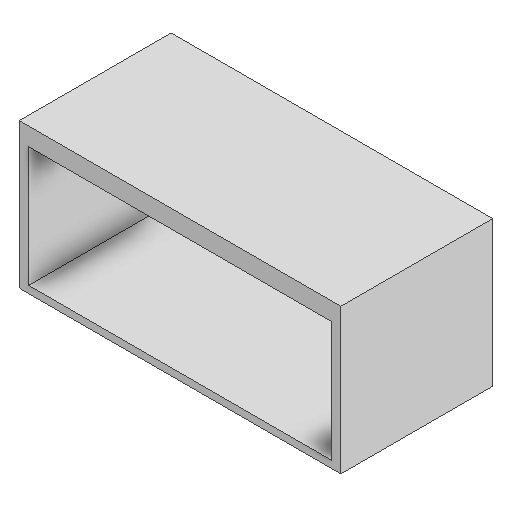
# Autodesk Inventor part: Liv Mas Base Box
Saved by Autodesk Inventor 2025.1 (Build 291241020, 241B)
## iProperties
Created: 2024-03-03
Part Number: Liv Mas Base Box
Material: Generic
Document SubType Name: Modeling
Designer: alexa_e021yt5
Density: 1 g/cm^3
Appearance: Default
Author: alexa_e021yt5
Autodesk Inventor part; units mm, degrees
ref_plane "YZ Plane" through (0, 0, 0) normal (1, 0, 0) x (0, 1, 0)
ref_plane "XZ Plane" through (0, 0, 0) normal (0, 1, 0) x (-1, 0, 0)
ref_plane "XY Plane" through (0, 0, 0) normal (0, 0, 1) x (1, 0, 0)
sketch "Sketch1" plane through (0, 0, 0) normal (0, 0, 1) x (1, 0, 0)
  line L0 (6.35, -116.84) -> (8.89, -119.38)
  line L1 (8.89, -119.38) -> (8.89, -121.92)
  line L2 (6.35, -84.074) -> (6.35, -116.84)
  line L3 (8.89, -81.534) -> (6.35, -84.074)
  line L4 (8.89, -68.58) -> (8.89, -81.534)
  line L5 (74.93, -68.58) -> (8.89, -68.58)
  line L6 (74.93, -121.92) -> (74.93, -68.58)
  line L7 (8.89, -121.92) -> (74.93, -121.92)
  line L8 (5.334, -117.2608) -> (7.874, -119.8008)
  line L9 (7.874, -119.8008) -> (7.874, -122.936)
  line L10 (7.874, -122.936) -> (75.946, -122.936)
  line L11 (75.946, -122.936) -> (75.946, -67.564)
  line L12 (75.946, -67.564) -> (7.874, -67.564)
  line L13 (7.874, -67.564) -> (7.874, -81.1132)
  line L14 (7.874, -81.1132) -> (5.334, -83.6532)
  line L15 (5.334, -83.6532) -> (5.334, -117.2608)
  line L16 (0, -63.5) -> (81.28, -63.5)
  line L17 (81.28, -63.5) -> (81.28, 0)
  line L18 (81.28, 0) -> (0, 0)
  line L19 (0, 0) -> (0, -63.5)
  line L20 (5.334, -111.1172) -> (0, -111.1172) construction
  line L21 (75.946, -101.4463) -> (81.28, -101.4463) construction
  line L22 (34.5139, -122.936) -> (34.5139, -63.5) construction
  line L23 (37.8868, -59.436) -> (37.8868, 0) construction
  line L24 (75.946, -76.28) -> (81.28, -76.28)
  line L25 (75.946, -120.595) -> (81.28, -120.595)
  line L26 (75.946, -107.895) -> (81.28, -107.895)
  line L27 (75.946, -91.52) -> (79.6093, -91.52)
  line L28 (81.28, -89.46) -> (81.28, -78.34)
  line L29 (76.835, -110.245) -> (76.835, -118.245)
  circle A0 centre (8.89, -114.3) radius 1.5875
  circle A1 centre (60.96, -119.38) radius 1.5875
  circle A2 centre (59.69, -71.12) radius 1.5875
  circle A3 centre (8.89, -86.36) radius 1.5875
  circle A4 centre (8.89, -114.3) radius 1.0795
  circle A5 centre (8.89, -86.36) radius 1.0795
  circle A6 centre (59.69, -71.12) radius 1.0795
  circle A7 centre (60.96, -119.38) radius 1.0795
  circle A8 centre (40.64, -95.2527) radius 8.89
  line L30 (6.35, -10.16) -> (8.89, -7.62)
  line L31 (8.89, -7.62) -> (8.89, -5.08)
  line L32 (6.35, -42.926) -> (6.35, -10.16)
  line L33 (8.89, -45.466) -> (6.35, -42.926)
  line L34 (8.89, -58.42) -> (8.89, -45.466)
  line L35 (74.93, -58.42) -> (8.89, -58.42)
  line L36 (74.93, -5.08) -> (74.93, -58.42)
  line L37 (8.89, -5.08) -> (74.93, -5.08)
  line L38 (5.334, -9.7392) -> (7.874, -7.1992)
  line L39 (7.874, -7.1992) -> (7.874, -4.064)
  line L40 (7.874, -4.064) -> (75.946, -4.064)
  line L41 (75.946, -4.064) -> (75.946, -59.436)
  line L42 (75.946, -59.436) -> (7.874, -59.436)
  line L43 (7.874, -59.436) -> (7.874, -45.8868)
  line L44 (7.874, -45.8868) -> (5.334, -43.3468)
  line L45 (5.334, -43.3468) -> (5.334, -9.7392)
  line L46 (5.334, -15.8828) -> (0, -15.8828) construction
  line L47 (75.946, -25.5537) -> (81.28, -25.5537) construction
  line L48 (75.946, -50.72) -> (81.28, -50.72)
  line L49 (75.946, -6.405) -> (81.28, -6.405)
  line L50 (75.946, -19.105) -> (81.28, -19.105)
  line L51 (75.946, -35.48) -> (81.28, -35.48)
  line L52 (81.28, -37.54) -> (81.28, -48.66)
  line L53 (76.835, -16.755) -> (76.835, -8.755)
  circle A9 centre (8.89, -12.7) radius 1.5875
  circle A10 centre (60.96, -7.62) radius 1.5875
  circle A11 centre (59.69, -55.88) radius 1.5875
  circle A12 centre (8.89, -40.64) radius 1.5875
  circle A13 centre (8.89, -12.7) radius 1.0795
  circle A14 centre (8.89, -40.64) radius 1.0795
  circle A15 centre (59.69, -55.88) radius 1.0795
  circle A16 centre (60.96, -7.62) radius 1.0795
  circle A17 centre (40.64, -31.7473) radius 8.89
  point P0 (0, 0)
  point P1 (81.28, -130.1977)
  point P2 (77.7776, -91.52)
  point P3 (81.28, -83.9)
  point P4 (76.835, -114.245)
  point P5 (8.89, -120.65)
  point P6 (41.91, -121.92)
  point P7 (81.28, 3.1977)
  point P8 (34.5139, -4.064)
  point P9 (79.6093, -35.48)
  point P10 (77.7776, -35.48)
  point P11 (81.28, -43.1)
  point P12 (76.835, -12.755)
  point P13 (8.89, -6.35)
  point P14 (41.91, -5.08)
  dimension "d0" = 1.016
  dimension "d1" = 81.28
  dimension "d2" = 63.5
  dimension "d3" = 15.24
  dimension "d4" = 7.62
  dimension "d5" = 12.7
  dimension "d6" = 6.35
  dimension "d7" = 2.159
  dimension "d8" = 2.159
  dimension "d9" = 2.159
  dimension "d10" = 2.159
  dimension "d38" = 17.78
  dimension "d40" = 40.64
  dimension "d93" = 5.334
  dimension "d94" = 63.5
  dimension "d96" = 55.372
  dimension "d97" = 4.064
  dimension "d98" = 4.6592
  dimension "d99" = 2.54
  dimension "d100" = 12.954
  dimension "d101" = 12.5332
  dimension "d102" = 15.0732
  dimension "d103" = 15.494
  dimension "d104" = 6.35
  dimension "d105" = 35.56
  dimension "d106" = 2.54
  dimension "d107" = 50.8
  dimension "d108" = 6.1261
  dimension "d109" = 1.27
  dimension "d110" = 26.6673
  constraints: 108 end point, 44 symmetric about line, 18 centre point, 16 point on line, 9 perpendicular, 5 midpoint, 4 parallel, 1 horizontal, 16 other
  measures "d0" distance between parallel lines of L15 L2
  measures "d1" distance between parallel lines of L17 L19
  measures "d2" distance between parallel lines of L16 L18
  measures "d3" distance from line of point (77.778, -91.52) L24
  measures "d4" distance from line of point (81.28, -83.9) L24
  measures "d5" distance between parallel lines of L25 L26
  measures "d6" distance from line of point (76.835, -114.245) L25
  measures "d7" diameter of A4
  measures "d8" diameter of A7
  measures "d9" diameter of A6
  measures "d10" diameter of A5
  measures "d38" diameter of A8
  measures "d40" distance from line of A8.centre L19
  measures "d93" distance of L20.start L20.end
  measures "d94" distance from line of point (0, 0) L16
  measures "d96" distance between parallel lines of L10 L12
  measures "d97" distance between parallel lines of L16 L12
  measures "d98" distance from line of L7 L8.start
  measures "d99" distance from line of L7 L0.end
  measures "d100" distance from line of L5 L3.start
  measures "d101" distance from line of L5 L13.end
  measures "d102" distance from line of L5 L14.end
  measures "d103" distance from line of L5 L2.start
  measures "d104" distance of point (8.89, -120.65) A0.centre
  measures "d105" distance from line of L7 A3.centre
  measures "d106" distance from line of L7 A1.centre
  measures "d107" distance from line of L7 A2.centre
  measures "d108" distance from line of L22 A8.centre
  measures "d109" horizontal distance of point (41.91, -121.92) A8.centre
  measures "d110" distance from line of L7 A8.centre
extrude "Extrusion1" add sketch "Sketch1" against normal blind 2.54 contours L19 L18 L17 L49 L41 L40 L39 L38 L45 L44 L43 L42 L48 L16 | L48 L41 L51 L17 | L41 L42 L43 L44 L45 L38 L39 L40 | L17 L50 L41 L49 | L41 L50 L17 L51 | L30 L31 L37 L36 L35 L34 L33 L32 | A9 | A10 | A11 | A12 | A13 | A14 | A15 | A16 | A17
extrude "Extrusion2" add sketch "Sketch1" along normal blind 7.62 contours L19 L18 L17 L49 L41 L40 L39 L38 L45 L44 L43 L42 L48 L16 | L41 L50 L17 L51 | A9 | A10 | A11 | A12 | A13 | A14 | A15 | A16
extrude "Extrusion4" add sketch "Sketch1" along normal blind 2.54 contours L19 L18 L17 L49 L41 L40 L39 L38 L45 L44 L43 L42 L48 L16 | L48 L41 L51 L17 | L17 L50 L41 L49 | L41 L50 L17 L51 | A9 | A10 | A11 | A12 | A13 | A14 | A15 | A16
sketch "Sketch9" plane through (0, 0, -2.54) normal (0, 0, -1) x (-1, 0, 0)
  line L0 (-81.28, -6.405) -> (-81.28, 0) projected
  line L1 (0, 0) -> (-81.28, 0)
  line L2 (-81.28, -63.5) -> (0, -63.5) projected
  line L3 (-81.28, 0) -> (-81.28, -63.5)
  line L4 (-81.28, -63.5) -> (-182.88, -63.5)
  line L5 (-182.88, -63.5) -> (-182.88, 19.05)
  line L6 (-182.88, 19.05) -> (0, 19.05)
  line L7 (0, 19.05) -> (0, 0)
  dimension "d115" = 182.88
  dimension "d116" = 19.05
  constraints: 12 end point, 5 perpendicular, 1 horizontal
  measures "d115" distance between parallel lines of L5 L7
  measures "d116" distance between parallel lines of L6 L1
extrude "Extrusion14" add sketch "Sketch9" against normal up to surface (10.16 mm away)
sketch "Sketch10" plane through (0, 0, 7.62) normal (0, 0, 1) x (1, 0, 0)
  line L0 (81.28, -19.105) -> (81.28, -6.405) projected
  line L1 (81.28, -50.72) -> (81.28, -35.48) projected
  line L2 (0, -63.5) -> (182.88, -63.5) projected
  line L3 (81.28, -6.405) -> (157.48, -6.405)
  line L4 (157.48, -6.405) -> (157.48, -63.5)
  line L5 (157.48, -63.5) -> (81.28, -63.5)
  line L6 (81.28, -63.5) -> (81.28, -6.405)
  point P0 (0, 0)
  dimension "d119" = 76.2
  constraints: 8 end point, 2 parallel, 1 horizontal, 1 perpendicular, 1 point on line
  measures "d119" distance between parallel lines of L0 L4
extrude "Extrusion15" cut sketch "Sketch10" against normal up to surface (7.62 mm away)
fillet "Fillet1" radius 38.1 1 edges at (157.48, -6.405, 3.81)
sketch "Sketch11" plane through (0, 19.05, -2.54) normal (0, 1, 0) x (1, 0, 0)
  line L0 (0, 0) -> (0, -10.16) projected
  line L1 (0, 0) -> (182.88, 0)
  line L2 (182.88, 0) -> (182.88, -86.36)
  line L3 (182.88, -86.36) -> (0, -86.36)
  line L4 (0, -86.36) -> (0, 0)
  line L5 (182.88, 0) -> (182.88, -10.16) projected
  line L6 (0, -10.16) -> (182.88, -10.16) projected
  point P0 (0, -2.54)
  dimension "d123" = 76.2
  constraints: 8 end point, 2 parallel, 1 horizontal, 1 perpendicular, 1 point on line
  measures "d123" distance between parallel lines of L3 L6
extrude "Extrusion16" add sketch "Sketch11" against normal blind 10.16 contours L6 L2 L3 L4
sketch "Sketch12" plane through (0, 8.89, -2.54) normal (0, -1, 0) x (1, 0, 0)
  line L0 (6.985, 77.47) -> (175.895, 77.47)
  line L1 (175.895, 77.47) -> (175.895, 19.05)
  line L2 (175.895, 19.05) -> (6.985, 19.05)
  line L3 (6.985, 19.05) -> (6.985, 77.47)
  line L4 (0, 86.36) -> (0, 10.16) projected
  line L5 (182.88, 86.36) -> (0, 86.36) projected
  point P0 (0, 2.54)
  point P1 (91.44, 77.47)
  point P2 (91.44, 86.36)
  point P3 (6.985, 48.26)
  point P4 (0, 48.26)
  dimension "d126" = 168.91
  dimension "d127" = 58.42
  constraints: 8 end point, 4 midpoint, 2 parallel, 1 horizontal, 1 horizontal alignment, 1 perpendicular, 1 vertical alignment
  measures "d126" distance of L0.start L0.end
  measures "d127" distance of L2.end L0.start
extrude "Extrusion17" cut sketch "Sketch12" against normal blind 5.08
sketch "Sketch13" plane through (0, 0, 7.62) normal (0, 0, 1) x (1, 0, 0)
  line L0 (182.88, 8.89) -> (0, 8.89) projected
  line L1 (5.334, 8.89) -> (5.334, -59.436)
  line L2 (5.334, -59.436) -> (177.546, -59.436)
  line L3 (177.546, -59.436) -> (177.546, 8.89)
  line L4 (182.88, 8.89) -> (182.88, -63.5) projected
  line L5 (0, -63.5) -> (0, 8.89) projected
  line L6 (0, -63.5) -> (81.28, -63.5) projected
  line L7 (157.48, -63.5) -> (81.28, -63.5) projected
  line L8 (157.48, -63.5) -> (182.88, -63.5) projected
  point P0 (0, 0)
  point P1 (7.874, -59.436)
  point P2 (5.334, -43.3468)
  point P3 (177.546, -25.273)
  dimension "d131" = 5.334
  constraints: 6 end point, 3 point on line, 2 perpendicular, 1 midpoint, 1 vertical
  measures "d131" distance from line of L4 point (177.546, -25.273)
extrude "Extrusion18" add sketch "Sketch13" along normal up to surface (76.2 mm away) contours L4 L8 L7 L6 L5 L0 L1 L2 L3
sketch "Sketch14" plane through (0, -63.5, -2.54) normal (0, -1, 0) x (1, 0, 0)
  line L0 (81.28, 10.16) -> (157.48, 10.16) projected
  line L1 (81.28, 5.08) -> (81.28, 10.16) projected
  line L2 (81.28, 10.16) -> (157.48, 10.16)
  line L3 (157.48, 10.16) -> (157.48, 21.59)
  line L4 (157.48, 21.59) -> (81.28, 21.59)
  line L5 (81.28, 21.59) -> (81.28, 10.16)
  line L6 (157.48, 2.54) -> (81.28, 2.54) projected
  point P0 (0, 2.54)
  dimension "d134" = 19.05
  constraints: 8 end point, 2 parallel, 1 horizontal, 1 perpendicular, 1 point on line
  measures "d134" distance between parallel lines of L4 L6
extrude "Extrusion19" cut sketch "Sketch14" against normal blind 20.6375
sketch "Sketch15" plane through (0, -63.5, -2.54) normal (0, -1, 0) x (1, 0, 0)
  line L0 (81.28, 21.59) -> (81.28, 10.16) projected
  line L1 (157.48, 2.54) -> (119.38, 2.54) projected
  line L2 (81.28, 21.59) -> (132.08, 21.59)
  line L3 (132.08, 21.59) -> (132.08, 2.54)
  line L4 (132.08, 2.54) -> (81.28, 2.54)
  line L5 (81.28, 2.54) -> (81.28, 21.59)
  line L6 (157.48, 21.59) -> (157.48, 2.54) projected
  point P0 (0, 2.54)
  dimension "d137" = 25.4
  constraints: 8 end point, 2 parallel, 1 horizontal, 1 perpendicular, 1 point on line
  measures "d137" distance between parallel lines of L6 L3
extrude "Extrusion20" add sketch "Sketch15" against normal up to surface (4.064 mm away)
sketch "Sketch16" plane through (0, -63.5, -2.54) normal (0, -1, 0) x (1, 0, 0)
  line L0 (82.6763, 9.3083) -> (61.6198, 9.2379)
  line L1 (61.6198, 9.2379) -> (51.0306, 27.4381)
  line L2 (51.0306, 27.4381) -> (61.4978, 45.7088)
  line L3 (61.4978, 45.7088) -> (82.5543, 45.7792)
  line L4 (82.5543, 45.7792) -> (93.1436, 27.579)
  line L5 (93.1436, 27.579) -> (82.6763, 9.3083)
  line L6 (64.5477, 40.4668) -> (57.0952, 27.4584)
  line L7 (57.0952, 27.4584) -> (64.6346, 14.5002)
  line L8 (64.6346, 14.5002) -> (79.6264, 14.5503)
  line L9 (79.6264, 14.5503) -> (87.0789, 27.5587)
  line L10 (87.0789, 27.5587) -> (79.5395, 40.5169)
  line L11 (79.5395, 40.5169) -> (64.5477, 40.4668)
  line L12 (51.0044, 35.8885) -> (50.9339, 56.9531)
  line L13 (50.9339, 56.9531) -> (56.2001, 56.9707)
  line L14 (56.2001, 56.9707) -> (56.24, 45.0273)
  line L15 (56.24, 45.0273) -> (51.0044, 35.8885)
  line L16 (61.4193, 71.0002) -> (66.6855, 71.0179)
  line L17 (66.6855, 71.0179) -> (66.7559, 49.9533)
  line L18 (82.5544, 50.0062) -> (82.4839, 71.0707)
  line L19 (82.4839, 71.0707) -> (77.2177, 71.0531)
  line L20 (77.2177, 71.0531) -> (77.2882, 49.9885)
  line L21 (93.1336, 35.9943) -> (93.063, 57.094)
  line L22 (93.063, 57.094) -> (87.7969, 57.0764)
  line L23 (87.7969, 57.0764) -> (87.837, 45.0979)
  line L24 (87.837, 45.0979) -> (93.1336, 35.9943)
  line L25 (69.3009, 76.2928) -> (69.389, 49.9621)
  line L26 (69.389, 49.9621) -> (74.6552, 49.9797)
  line L27 (74.6552, 49.9797) -> (74.5671, 76.3104)
  line L28 (74.5671, 76.3104) -> (69.3009, 76.2928)
  line L29 (77.2882, 49.9885) -> (82.5544, 50.0062)
  line L30 (66.6855, 71.0179) -> (69.3185, 71.0267) construction
  line L31 (77.2177, 71.0531) -> (74.5847, 71.0443) construction
  line L32 (61.4193, 71.0002) -> (61.4898, 49.9357)
  line L33 (61.4898, 49.9357) -> (66.7559, 49.9533)
  point P0 (0, 2.54)
  point P1 (72.0871, 27.5085)
  point P2 (95.9605, 86.1193)
  dimension "d140" = 21.0566
  dimension "d141" = 5.2522
  dimension "d142" = 4.2234
  dimension "d143" = 4.2234
  dimension "d144" = 5.2662
  dimension "d145" = 5.2662
  dimension "d146" = 5.2662
  dimension "d147" = 5.2662
  dimension "d148" = 4.2269
  dimension "d149" = 21.0647
  dimension "d150" = 21.0647
  dimension "d151" = 26.3309
  dimension "d152" = 5.2662
  dimension "d153" = 5.2662
  dimension "d154" = 5.2662
  dimension "d155" = 2.6331
  dimension "d156" = 5.2578
  constraints: 68 end point, 8 perpendicular, 7 point on line, 5 parallel, 3 collinear, 18 other
  measures "d140" distance of L0.start L1.start
  measures "d141" distance between parallel lines of L2 L6
  measures "d142" distance between parallel lines of L15 L2
  measures "d143" distance between parallel lines of L24 L4
  measures "d144" distance between parallel lines of L14 L12
  measures "d145" distance between parallel lines of L21 L23
  measures "d146" distance between parallel lines of L18 L20
  measures "d147" distance between parallel lines of L25 L27
  measures "d148" distance between parallel lines of L33 L3
  measures "d149" distance between parallel lines of L16 L33
  measures "d150" distance from line of L13 L12.start
  measures "d151" distance between parallel lines of L28 L26
  measures "d152" distance between parallel lines of L32 L17
  measures "d153" distance between parallel lines of L32 L14
  measures "d154" distance between parallel lines of L23 L18
  measures "d155" distance between parallel lines of L27 L20
  measures "d156" horizontal distance of L3.start L15.start
extrude "Extrusion21" add sketch "Sketch16" along normal blind 2.54
chamfer "Chamfer3" distance 2.54 angle 45 11 edges at (90.4853, -66.04, 38.0061) (79.9213, -66.04, 47.4573) (72.0221, -66.04, 47.4309) (64.1229, -66.04, 47.4045) (53.6222, -66.04, 37.9179) (56.3252, -66.04, 15.798) (72.1481, -66.04, 6.7331) (87.9099, -66.04, 15.9036) (83.3092, -66.04, 31.4978) (72.0436, -66.04, 37.9518) (60.8215, -66.04, 31.4226)
equation "\"d4\" = 0.5 * d3"
equation "\"d6\" = 0.5 * d5"
equation "\"d8\" = d7"
equation "\"d9\" = d7"
equation "\"d10\" = d7"
body "Solid1"
